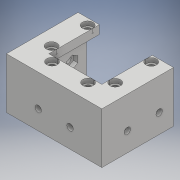
# Autodesk Inventor part: april_tag
Saved by Autodesk Inventor 2018 (Build 220112000, 112)
## iProperties
Created: 2018-06-13
Part Number: april_tag
Material: Generic
Document SubType Name: Modeling
Designer: bitbots
Density: 1 g/cm^3
Appearance: Default
Author: bitbots
Autodesk Inventor part; units mm, degrees
ref_plane "YZ Plane" through (0, 0, 0) normal (1, 0, 0) x (0, 1, 0)
ref_plane "Work Plane1" through (0, 0, 0) normal (0, 0, 1) x (1, 0, 0)
sketch "Sketch1" plane through (0, 0, 0) normal (0, 0, 1) x (1, 0, 0)
  line L0 (-12.7, 12) -> (-9.2, 12) construction
  line L1 (-12.7, 12) -> (-17.8, 6) construction
  line L2 (-17.8, 6) -> (-17.8, -32.6) construction
  line L3 (-17.8, -32.6) -> (-12.7, -38.6) construction
  line L4 (-12.7, -38.6) -> (12.7, -38.6) construction
  line L5 (12.7, -38.6) -> (17.8, -32.6) construction
  line L6 (17.8, -32.6) -> (17.8, 6) construction
  line L7 (17.8, 6) -> (12.7, 12) construction
  line L8 (9.2, 12) -> (12.7, 12) construction
  arc A0 (12.2, 9) -> (9.2, 12) centre (9.2, 9) ccw construction
  line L9 (12.2, -30) -> (12.2, 9) construction
  arc A1 (9.2, -33) -> (12.2, -30) centre (9.2, -30) ccw construction
  line L10 (-9.2, -33) -> (9.2, -33) construction
  arc A2 (-12.2, -30) -> (-9.2, -33) centre (-9.2, -30) ccw construction
  line L11 (-12.2, 9) -> (-12.2, -30) construction
  arc A3 (-9.2, 12) -> (-12.2, 9) centre (-9.2, 9) ccw construction
  circle A4 centre (-15, 4.5) radius 1.35 construction
  circle A5 centre (-15, -12.5) radius 1.35 construction
  circle A6 centre (-8.5, -35.8) radius 1.35 construction
  circle A7 centre (15, 4.5) radius 1.35 construction
  circle A8 centre (15, -12.5) radius 1.35 construction
  circle A9 centre (8.5, -35.8) radius 1.35 construction
  circle A10 centre (-15, -29.5) radius 1.35 construction
  circle A11 centre (15, -29.5) radius 1.35 construction
  line L12 (-15, -12.5) -> (-12.5, -12.5) construction
  line L13 (-12.5, -12.5) -> (-12.5, -9.5) construction
  line L14 (-12.5, -9.5) -> (-15, -9.5) construction
  line L15 (-15, -9.5) -> (-15, -12.5) construction
  line L16 (15, -12.5) -> (12.5, -12.5) construction
  line L17 (12.5, -12.5) -> (12.5, -9.5) construction
  line L18 (12.5, -9.5) -> (15, -9.5) construction
  line L19 (15, -9.5) -> (15, -12.5) construction
  line L20 (-8.5, -35.8) -> (-12.5, -35.8) construction
  line L21 (-12.5, -35.8) -> (-12.5, -33.3) construction
  line L22 (-12.5, -33.3) -> (-8.5, -33.3) construction
  line L23 (-8.5, -33.3) -> (-8.5, -35.8) construction
  line L24 (8.5, -35.8) -> (12.5, -35.8) construction
  line L25 (12.5, -35.8) -> (12.5, -33.3) construction
  line L26 (12.5, -33.3) -> (8.5, -33.3) construction
  line L27 (8.5, -33.3) -> (8.5, -35.8) construction
  line L28 (-12.5, -9.5) -> (-22.5, -9.5)
  line L29 (-22.5, -9.5) -> (-22.5, -33.3)
  line L30 (-22.5, -33.3) -> (-12.5, -33.3)
  line L31 (-12.5, -33.3) -> (-12.5, -9.5)
  line L32 (12.5, -9.5) -> (22.5, -9.5)
  line L33 (22.5, -9.5) -> (22.5, -33.3)
  line L34 (22.5, -33.3) -> (12.5, -33.3)
  line L35 (12.5, -33.3) -> (12.5, -9.5)
  line L36 (-22.5, -33.3) -> (22.5, -33.3)
  line L37 (22.5, -33.3) -> (22.5, -43.3)
  line L38 (22.5, -43.3) -> (-22.5, -43.3)
  line L39 (-22.5, -43.3) -> (-22.5, -33.3)
  circle A12 centre (-15, -12.5) radius 1.5
  circle A13 centre (-15, -29.5) radius 1.5
  circle A14 centre (-8.5, -35.8) radius 1.5
  circle A15 centre (8.5, -35.8) radius 1.5
  circle A16 centre (15, -29.5) radius 1.5
  circle A17 centre (15, -12.5) radius 1.5
  point P0 (0, 0)
  dimension "d0" = 2.5
  dimension "d1" = 3
  dimension "d2" = 2.5
  dimension "d3" = 3
  dimension "d4" = 4
  dimension "d5" = 2.5
  dimension "d6" = 4
  dimension "d7" = 2.5
  dimension "d9" = 10
  dimension "d10" = 10
  dimension "d11" = 10
  dimension "d12" = 3
  dimension "d13" = 3
  dimension "d14" = 3
  dimension "d15" = 3
  dimension "d16" = 3
  dimension "d17" = 3
  constraints: 56 end point, 14 parallel, 7 horizontal, 7 perpendicular, 6 centre point, 6 coincident, 2 point on line
  measures "d0" distance of L14.end L13.end
  measures "d1" distance of L13.end L12.end
  measures "d2" distance of L17.end L18.end
  measures "d3" distance of L16.end L17.end
  measures "d4" distance of L21.end L22.end
  measures "d5" distance of L20.end L21.end
  measures "d6" distance of L26.end L25.end
  measures "d7" distance of L25.end L24.end
  measures "d9" distance of L30.end L29.end
  measures "d10" distance of L33.end L34.end
  measures "d11" distance of L36.end L37.end
  measures "d12" diameter of A12
  measures "d13" diameter of A13
  measures "d14" diameter of A14
  measures "d15" diameter of A15
  measures "d16" diameter of A16
  measures "d17" diameter of A17
extrude "Extrusion1" add sketch "Sketch1" along normal blind 2
sketch "Sketch2" plane through (-22.5, -43.3, 0) normal (0, -1, 0) x (1, 0, 0)
  line L0 (0, 0) -> (45, 0) projected
  line L1 (45, 0) -> (45, 2) projected
  line L2 (0, 2) -> (45, 2) projected
  line L3 (0, 0) -> (0, 2) projected
  line L4 (0, 0) -> (45, 0)
  line L5 (45, 0) -> (45, -20)
  line L6 (45, -20) -> (0, -20)
  line L7 (0, -20) -> (0, 0)
  point P0 (22.5, 0)
  dimension "d20" = 20
  constraints: 8 end point, 2 parallel, 1 horizontal, 1 perpendicular
  measures "d20" distance of L4.end L5.end
extrude "Extrusion2" add sketch "Sketch2" against normal blind 4
ref_plane "Work Plane2" through (0, -43.3, 2) normal (-1, 0, 0) x (0, 0, 1)
sketch "Sketch3" plane through (-22.5, -43.3, 2) normal (-1, 0, 0) x (0, 0, 1)
  line L0 (0, 33.8) -> (0, 0) projected
  line L1 (-2, 33.8) -> (0, 33.8) projected
  line L2 (-2, 33.8) -> (-2, 4) projected
  line L3 (-22, 4) -> (-2, 4) projected
  line L4 (-22, 0) -> (-22, 4) projected
  line L5 (-22, 0) -> (0, 0) projected
  line L6 (-2, 33.8) -> (-2, 4) projected
  line L7 (-2, 4) -> (-22, 4)
  line L8 (-22, 4) -> (-22, 33.8)
  line L9 (-22, 33.8) -> (-2, 33.8)
  line L10 (-2, 33.8) -> (-2, 4)
  point P0 (-2, 43.3)
  constraints: 8 end point, 2 parallel, 1 horizontal, 1 perpendicular
extrude "Extrusion3" add sketch "Sketch3" against normal blind 4
mirror "Mirror1" about plane through (0, -43.3, 2) normal (-1, 0, 0) of "Extrusion3"
sketch "Sketch4" plane through (0, 0, 2) normal (0, 0, 1) x (1, 0, 0)
  line L0 (22.5, -9.5) -> (12.5, -9.5) projected
  line L1 (12.5, -9.5) -> (12.5, -33.3) projected
  line L2 (12.5, -33.3) -> (-12.5, -33.3) projected
  line L3 (-12.5, -33.3) -> (-12.5, -9.5) projected
  line L4 (-12.5, -9.5) -> (-22.5, -9.5) projected
  line L5 (-22.5, -9.5) -> (-22.5, -43.3) projected
  line L6 (-22.5, -43.3) -> (22.5, -43.3) projected
  line L7 (22.5, -43.3) -> (22.5, -9.5) projected
  circle A0 centre (8.5, -35.8) radius 1.5 projected
  circle A1 centre (-8.5, -35.8) radius 1.5 projected
  circle A2 centre (15, -12.5) radius 1.5 projected
  circle A3 centre (15, -29.5) radius 1.5 projected
  circle A4 centre (-15, -29.5) radius 1.5 projected
  circle A5 centre (-15, -12.5) radius 1.5 projected
  circle A6 centre (8.5, -35.8) radius 2.5
  circle A7 centre (15, -29.5) radius 1.5 projected
  circle A8 centre (15, -29.5) radius 2.5
  circle A9 centre (15, -12.5) radius 2.5
  circle A10 centre (-8.5, -35.8) radius 2.5
  circle A11 centre (-15, -29.5) radius 1.5 projected
  circle A12 centre (-15, -29.5) radius 2.5
  circle A13 centre (-15, -12.5) radius 2.5
  point P0 (0, 0)
  dimension "d25" = 5
  dimension "d26" = 5
  dimension "d27" = 5
  dimension "d28" = 5
  dimension "d29" = 5
  dimension "d30" = 5
  constraints: 6 centre point, 6 coincident
  measures "d25" diameter of A6
  measures "d26" diameter of A8
  measures "d27" diameter of A9
  measures "d28" diameter of A10
  measures "d29" diameter of A12
  measures "d30" diameter of A13
extrude "Extrusion4" add sketch "Sketch4" along normal blind 2 contours L7 L6 L5 L4 L3 L2 L1 L0
sketch "Sketch5" plane through (-22.5, -43.3, -20) normal (0, -1, 0) x (1, 0, 0)
  line L0 (0, 0) -> (0, 24) construction
  line L1 (0, 0) -> (45, 0) construction
  line L2 (45, 0) -> (45, 24) construction
  line L3 (0, 24) -> (45, 24) construction
  line L4 (0, 24) -> (15, 24) construction
  line L5 (15, 24) -> (15, 9) construction
  line L6 (15, 9) -> (0, 9) construction
  line L7 (0, 9) -> (0, 24) construction
  line L8 (15, 9) -> (30, 9) construction
  circle A0 centre (15, 9) radius 1.5
  circle A1 centre (30, 9) radius 1.5
  point P0 (22.5, 20)
  dimension "d33" = 15
  dimension "d34" = 15
  dimension "d35" = 15
  dimension "d36" = 3
  dimension "d37" = 3
  constraints: 10 end point, 2 centre point, 2 coincident, 2 horizontal, 2 parallel, 1 perpendicular
  measures "d33" distance of L5.end L6.end
  measures "d34" distance of L4.end L5.end
  measures "d35" distance of L5.end L8.end
  measures "d36" diameter of A0
  measures "d37" diameter of A1
extrude "Extrusion5" cut sketch "Sketch5" against normal through all
sketch "Sketch6" plane through (-22.5, -39.3, 0) normal (0, 1, 0) x (1, 0, 0)
  circle A0 centre (15, 11) radius 1.5 projected
  circle A1 centre (30, 11) radius 1.5 projected
  line L0 (41, 0) -> (41, 20) projected
  line L1 (41, 20) -> (4, 20) projected
  line L2 (4, 20) -> (4, 0) projected
  line L3 (41, 0) -> (4, 0) projected
  line L4 (15, 11) -> (17.6, 11)
  line L5 (17.6, 9.4989) -> (15, 7.9978)
  line L6 (15, 7.9978) -> (12.4, 9.4989)
  line L7 (12.4, 9.4989) -> (12.4, 12.5011)
  line L8 (12.4, 12.5011) -> (15, 14.0022)
  line L9 (15, 14.0022) -> (17.6, 12.5011)
  line L10 (17.6, 12.5011) -> (17.6, 9.4989)
  line L11 (30, 11) -> (32.6, 11)
  line L12 (32.6, 9.4989) -> (30, 7.9978)
  line L13 (30, 7.9978) -> (27.4, 9.4989)
  line L14 (27.4, 9.4989) -> (27.4, 12.5011)
  line L15 (27.4, 12.5011) -> (30, 14.0022)
  line L16 (30, 14.0022) -> (32.6, 12.5011)
  line L17 (32.6, 12.5011) -> (32.6, 9.4989)
  point P0 (22.5, 0)
  dimension "d40" = 2.6
  dimension "d41" = 2.6
  constraints: 28 end point, 2 coincident, 2 horizontal, 2 midpoint, 26 other
  measures "d40" distance of L4.start L4.end
  measures "d41" distance of L11.start L11.end
extrude "Extrusion6" cut sketch "Sketch6" against normal blind 2 contours L10 L5 L6 L7 L8 L9 | L17 L12 L13 L14 L15 L16
sketch "Sketch7" plane through (-22.5, -43.3, -20) normal (-1, 0, 0) x (0, 0, 1)
  line L0 (0, 33.8) -> (24, 33.8) construction
  line L1 (0, 0) -> (0, 33.8) construction
  line L2 (0, 0) -> (24, 0) construction
  line L3 (24, 33.8) -> (24, 0) construction
  line L4 (0, 33.8) -> (10, 33.8) construction
  line L5 (10, 33.8) -> (10, 28.8) construction
  line L6 (10, 28.8) -> (0, 28.8) construction
  line L7 (0, 28.8) -> (0, 33.8) construction
  line L8 (0, 0) -> (0, 33.8) construction
  line L9 (0, 0) -> (9, 0) construction
  line L10 (9, 0) -> (9, 12) construction
  line L11 (9, 12) -> (0, 12) construction
  line L12 (0, 12) -> (0, 0) construction
  line L13 (9, 12) -> (9, 27) construction
  circle A0 centre (9, 27) radius 1.5
  circle A1 centre (9, 12) radius 1.5
  point P0 (20, 43.3)
  dimension "d44" = 10
  dimension "d45" = 5
  dimension "d46" = 9
  dimension "d47" = 12
  dimension "d48" = 15
  dimension "d49" = 3
  dimension "d50" = 3
  constraints: 18 end point, 4 parallel, 2 centre point, 2 coincident, 2 horizontal, 2 perpendicular, 1 vertical
  measures "d44" distance of L5.end L6.end
  measures "d45" distance of L4.end L5.end
  measures "d46" distance of L11.end L10.end
  measures "d47" distance of L10.end L9.end
  measures "d48" distance of L10.end L13.end
  measures "d49" diameter of A0
  measures "d50" diameter of A1
extrude "Extrusion7" cut sketch "Sketch7" against normal through all
sketch "Sketch8" plane through (-18.5, -43.3, 2) normal (1, 0, 0) x (0, 0, -1)
  circle A0 centre (13, 27) radius 1.5 construction
  circle A1 centre (13, 12) radius 1.5 construction
  line L0 (22, 4) -> (2, 4) construction
  line L1 (22, 4) -> (22, 33.8) construction
  line L2 (22, 33.8) -> (2, 33.8) construction
  line L3 (2, 4) -> (2, 33.8) construction
  line L4 (13, 12) -> (13, 14.6) construction
  line L5 (14.5011, 14.6) -> (16.0022, 12)
  line L6 (16.0022, 12) -> (14.5011, 9.4)
  line L7 (14.5011, 9.4) -> (11.4989, 9.4)
  line L8 (11.4989, 9.4) -> (9.9978, 12)
  line L9 (9.9978, 12) -> (11.4989, 14.6)
  line L10 (11.4989, 14.6) -> (14.5011, 14.6)
  circle A2 centre (13, 27) radius 1.5 projected
  line L11 (13, 27) -> (13, 29.6)
  line L12 (14.5011, 29.6) -> (16.0022, 27)
  line L13 (16.0022, 27) -> (14.5011, 24.4)
  line L14 (14.5011, 24.4) -> (11.4989, 24.4)
  line L15 (11.4989, 24.4) -> (9.9978, 27)
  line L16 (9.9978, 27) -> (11.4989, 29.6)
  line L17 (11.4989, 29.6) -> (14.5011, 29.6)
  point P0 (2, 43.3)
  dimension "d53" = 2.6
  dimension "d54" = 2.6
  constraints: 28 end point, 2 coincident, 2 midpoint, 2 vertical, 26 other
  measures "d53" distance of L4.start L4.end
  measures "d54" distance of L11.start L11.end
extrude "Extrusion8" cut sketch "Sketch8" against normal blind 2
mirror "Mirror2" about plane through (0, -43.3, 2) normal (-1, 0, 0) of "Extrusion8"
body "Solid1"
